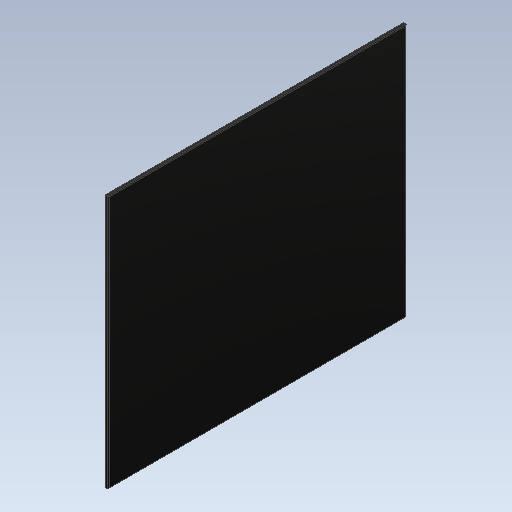
# Autodesk Inventor part: solar3
Saved by Autodesk Inventor 2020 (Build 240168000, 168)
## iProperties
Created: 2017-11-20
Part Number: solar3
Material: Generic
Document SubType Name: Modeling
Designer: stedrock
Density: 1 g/cm^3
Appearance: Default
Mass: 67.9603 g
Surface Area: 693.211 cm^2
Volume: 67.9603 cm^3
Author: stedrock
Autodesk Inventor part; units mm, degrees
ref_plane "YZ Plane" through (0, 0, 0) normal (1, 0, 0) x (0, 1, 0)
ref_plane "XZ Plane" through (0, 0, 0) normal (0, 1, 0) x (-1, 0, 0)
ref_plane "XY Plane" through (0, 0, 0) normal (0, 0, 1) x (1, 0, 0)
sketch "Sketch1" plane through (0, 0, 0) normal (1, 0, 0) x (0, 1, 0)
  line L0 (-85, 100) -> (85, 100)
  line L1 (85, 100) -> (85, -100)
  line L2 (85, -100) -> (-85, -100)
  line L3 (-85, -100) -> (-85, 100)
  line L4 (-85, 100) -> (85, -100) construction
  line L5 (85, 100) -> (-85, -100) construction
  point P0 (0, 0)
  dimension "d0" = 170
  dimension "d1" = 200
  constraints: 12 end point, 2 midpoint, 2 parallel, 1 horizontal, 1 perpendicular
  measures "d0" distance of L1.end L2.end
  measures "d1" distance of L0.end L1.end
extrude "Extrusion1" add sketch "Sketch1" along normal blind 2
fillet "Fillet1" radius 0.5 4 edges at (2, -85, 0) (2, 0, -100) (2, 85, 0) (2, 0, 100)
body "Solid1"
